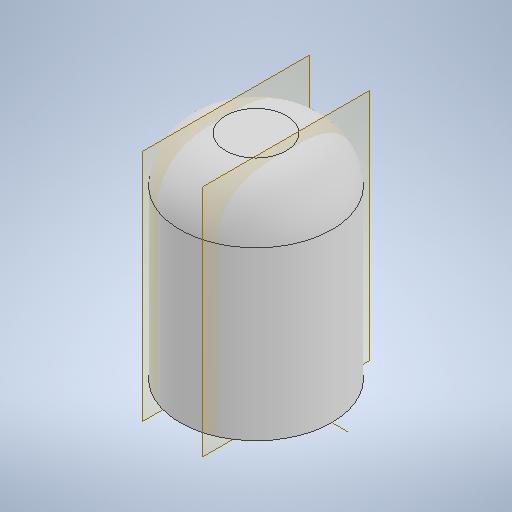
# Autodesk Inventor part: Base
Saved by Autodesk Inventor 2025.2 (Build 292293000, 293)
## iProperties
Created: 2025-02-16
Part Number: Base
Material: Generic
Document SubType Name: Modeling
Designer: eason
Density: 1 g/cm^3
Appearance: Default
Author: eason
Autodesk Inventor part; units mm, degrees
ref_plane "XZ Plane" through (0, 0, 0) normal (0, 1, 0) x (-1, 0, 0)
ref_plane "XY Plane" through (0, 0, 0) normal (0, 0, 1) x (1, 0, 0)
sketch "Sketch1" plane through (0, 0, 0) normal (0, 0, 1) x (1, 0, 0)
  line L0 (0, 0) -> (0, 70)
  line L1 (0, 0) -> (25, 0)
  line L2 (25, 0) -> (25, 55)
  line L3 (0, -14.6213) -> (0, 87.7279) projected
  line L4 (0, 70) -> (10, 70)
  arc A0 (25, 55) -> (10, 70) centre (10, 55) ccw
  dimension "d0" = 70
  dimension "d1" = 25
  dimension "d2" = 10
  constraints: 8 end point, 2 point on circle, 2 tangent, 2 vertical, 1 centre point, 1 horizontal, 1 perpendicular
  measures "d0" distance of L0.start L0.end
  measures "d1" distance of L0.start L1.end
  measures "d2" distance of L0.end L4.end
revolve "Revolution1" add sketch "Sketch1" angle 360 about axis through (0, -10, 0) along (0, 1, 0)
sketch "Sketch2" plane through (0, 0, 0) normal (0, -1, 0) x (1, 0, 0)
  circle A0 centre (0, 0) radius 10
  dimension "d4" = 20
  constraints: 1 centre point, 1 coincident
  measures "d4" diameter of A0
extrude "Extrusion1" cut sketch "Sketch2" against normal blind 25
sketch "Sketch3" plane through (0, 70, 0) normal (0, 1, 0) x (1, 0, 0)
  circle A0 centre (0, 0) radius 10 projected
  line L0 (10, 0) -> (-10, 0) construction
  line L1 (-35, 0) -> (35, 0) construction
  constraints: 2 end point, 2 point on circle, 1 collinear
ref_plane "Work Plane1" through (10, 70, 0) normal (1, 0, 0) x (0, 1, 0)
ref_plane "Work Plane2" through (-10, 70, 0) normal (1, 0, 0) x (0, 1, 0)
body "Solid1"
